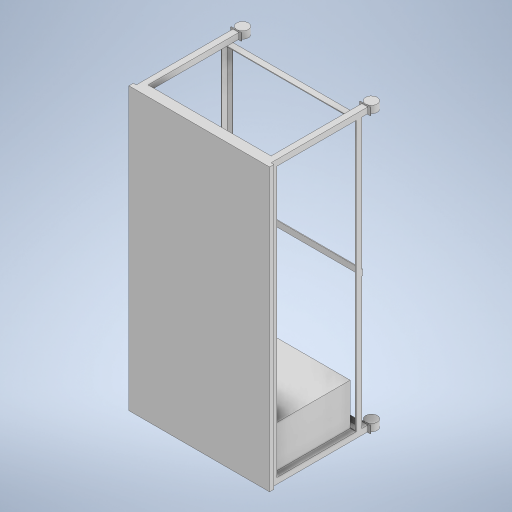
# Autodesk Inventor part: Table Model
Saved by Autodesk Inventor 2023 (Build 270158000, 158)
## iProperties
Created: 2022-09-16
Part Number: Table Model
Material: Generic
Document SubType Name: Modeling
Designer: mikep
Density: 1 g/cm^3
Appearance: Default
Mass: 146789 g
Surface Area: 91872.9 cm^2
Volume: 146789 cm^3
Author: mikep
Autodesk Inventor part; units mm, degrees
ref_plane "YZ Plane" through (0, 0, 0) normal (1, 0, 0) x (0, 1, 0)
ref_plane "XZ Plane" through (0, 0, 0) normal (0, 1, 0) x (-1, 0, 0)
ref_plane "XY Plane" through (0, 0, 0) normal (0, 0, 1) x (1, 0, 0)
sketch "Sketch1" plane through (0, 0, 0) normal (0, 0, 1) x (1, 0, 0)
  line L0 (0, 0) -> (1219.2, 0)
  line L1 (1219.2, 0) -> (1219.2, 2438.4)
  line L2 (1219.2, 2438.4) -> (0, 2438.4)
  line L3 (0, 2438.4) -> (0, 0)
  line L4 (609.6, 0) -> (609.6, 2438.4)
  dimension "d0" = 1219.2
  constraints: 10 end point, 2 midpoint, 2 parallel, 1 horizontal, 1 perpendicular
  measures "d0" distance of L2.end L1.end
extrude "Extrusion1" add sketch "Sketch1" along normal blind 38.1
sketch "Sketch2" plane through (0, 0, 0) normal (0, 0, -1) x (-1, 0, 0)
  line L0 (0, 2438.4) -> (0, 0) projected
  line L1 (-1219.2, 2438.4) -> (0, 2438.4) projected
  line L2 (0, 0) -> (0, 2438.4)
  line L3 (0, 2438.4) -> (-1219.2, 2438.4)
  line L4 (-1219.2, 0) -> (-1219.2, 2438.4) projected
  line L5 (-1219.2, 2438.4) -> (-1219.2, 0)
  line L6 (0, 0) -> (-1219.2, 0) projected
  line L7 (-1219.2, 0) -> (0, 0)
  line L8 (-76.2, 50.8) -> (-1143, 50.8)
  line L9 (-76.2, 50.8) -> (-76.2, 2387.6)
  line L10 (-76.2, 2387.6) -> (-1143, 2387.6)
  line L11 (-1143, 2387.6) -> (-1143, 50.8)
  line L12 (-76.2, 1193.8) -> (-1143, 1193.8)
  line L13 (-1143, 1244.6) -> (-76.2, 1244.6)
  line L14 (-25.4, 0) -> (-25.4, 2438.4)
  line L15 (-1193.8, 2438.4) -> (-1193.8, 0)
  point P0 (-609.6, 0)
  point P1 (-1193.8, 0)
  point P2 (-25.4, 2438.4)
  dimension "d4" = 50.8
  dimension "d5" = 1066.8
  dimension "d8" = 50.8
  dimension "d9" = 1193.8
  dimension "d11" = 50.8
  dimension "d13" = 25.4
  dimension "d19" = 50.8
  constraints: 24 end point, 8 point on line, 6 perpendicular, 3 collinear, 2 parallel, 1 midpoint, 1 vertical
  measures "d4" distance between parallel lines of L6 L8
  measures "d5" distance of L9.end L10.end
  measures "d8" distance between parallel lines of L12 L13
  measures "d9" distance from line of point (-609.6, 0) L12
  measures "d11" distance between parallel lines of L9 L14
  measures "d13" distance between parallel lines of L0 L14
  measures "d19" distance between parallel lines of L1 L10
extrude "Extrusion2" add sketch "Sketch2" along normal blind 50.8 contours L14 L6 L15 L1 | L12 L11 L13 L9
sketch "Sketch3" plane through (0, 0, -50.8) normal (0, 0, -1) x (-1, 0, 0)
  line L0 (-25.4, 2438.4) -> (-25.4, 0) projected
  line L1 (-76.2, 50.8) -> (-25.4, 50.8)
  line L2 (-25.4, 50.8) -> (-25.4, 0)
  line L3 (-25.4, 0) -> (-76.2, 0)
  line L4 (-76.2, 0) -> (-76.2, 50.8)
  line L5 (-1193.8, 0) -> (-25.4, 0) projected
  line L6 (-1143, 1193.8) -> (-1143, 50.8) projected
  line L7 (-1193.8, 0) -> (-1143, 0)
  line L8 (-1143, 0) -> (-1143, 50.8)
  line L9 (-1143, 50.8) -> (-1193.8, 50.8)
  line L10 (-1193.8, 50.8) -> (-1193.8, 0)
  line L11 (-1143, 2387.6) -> (-76.2, 2387.6) projected
  line L12 (-1143, 2387.6) -> (-1193.8, 2387.6)
  line L13 (-1193.8, 2387.6) -> (-1193.8, 2438.4)
  line L14 (-1193.8, 2438.4) -> (-1143, 2438.4)
  line L15 (-1143, 2438.4) -> (-1143, 2387.6)
  line L16 (-1219.2, 2438.4) -> (0, 2438.4) projected
  line L17 (-76.2, 2387.6) -> (-25.4, 2387.6)
  line L18 (-25.4, 2387.6) -> (-25.4, 2438.4)
  line L19 (-25.4, 2438.4) -> (-76.2, 2438.4)
  line L20 (-76.2, 2438.4) -> (-76.2, 2387.6)
  line L21 (-76.2, 1193.8) -> (-1143, 1193.8) projected
  point P0 (0, 0)
  point P1 (-25.4, 1244.6)
  dimension "d18" = 50.8
  constraints: 32 end point, 8 parallel, 6 point on line, 4 horizontal, 4 perpendicular
  measures "d18" distance of L14.end L11.start
extrude "Extrusion3" add sketch "Sketch3" along normal blind 736.6 contours L5 L10 L9 L8 | L0 L3 L4 L1 | L0 L17 L20 L16 | L15 L12 L13 L14
sketch "Sketch8" plane through (25.4, 2387.6, -50.8) normal (0, -1, 0) x (1, 0, 0)
  line L0 (0, -735.9482) -> (0, -685.1482)
  line L1 (0, 0) -> (0, -736.6) projected
  line L2 (0, -685.1482) -> (6.35, -685.1482)
  line L3 (50.8, -736.6) -> (0, -736.6) projected
  line L4 (0, -736.6) -> (50.8, -736.6)
  line L5 (50.8, -736.6) -> (50.8, -730.25)
  line L6 (50.8, 0) -> (50.8, -736.6) projected
  line L7 (50.8, -730.25) -> (6.35, -730.25)
  line L8 (6.35, -730.25) -> (6.35, -685.1482)
  line L9 (1168.4, 0) -> (1168.4, -736.6) projected
  line L10 (1168.4, -736.6) -> (1168.4, -685.8)
  line L11 (1168.4, -685.8) -> (1168.4, -736.6)
  line L12 (1168.4, -736.6) -> (1117.6, -736.6) projected
  line L13 (1168.4, -736.6) -> (1117.6, -736.6)
  line L14 (1117.6, -736.6) -> (1117.6, -730.25)
  line L15 (1117.6, 0) -> (1117.6, -736.6) projected
  line L16 (1117.6, -730.25) -> (1162.05, -730.25)
  line L17 (1162.05, -730.25) -> (1162.05, -685.8)
  line L18 (1162.05, -685.8) -> (1168.4, -685.8)
  point P0 (-25.4, 50.8)
  point P1 (0, -735.9482)
  dimension "d40" = 50.8
  dimension "d41" = 6.35
  dimension "d42" = 6.35
  dimension "d43" = 44.45
  dimension "d44" = 50.8
  dimension "d45" = 6.35
  dimension "d46" = 44.45
  dimension "d47" = 44.45
  constraints: 26 end point, 5 perpendicular, 4 point on line, 2 horizontal, 1 collinear
  measures "d40" distance of L0.start L0.end
  measures "d41" distance of L0.end L2.end
  measures "d42" distance of L3.start L5.end
  measures "d43" distance of L5.end L7.end
  measures "d44" distance of L9.end L10.end
  measures "d45" distance of L12.end L14.end
  measures "d46" distance of L14.end L16.end
  measures "d47" distance of L16.end L17.end
extrude "Extrusion6" add sketch "Sketch8" along normal blind 2336.8
sketch "Sketch9" plane through (1187.45, 50.8, -781.05) normal (-1, 0, 0) x (0, 0, 1)
  line L0 (44.45, 0) -> (0, 0) projected
  line L1 (44.45, 0) -> (44.45, 6.35)
  line L2 (44.45, 2336.8) -> (44.45, 0) projected
  line L3 (44.45, 6.35) -> (0, 6.35)
  line L4 (0, 2336.8) -> (0, 0) projected
  line L5 (44.45, 2336.8) -> (44.45, 0) projected
  line L6 (0, 0) -> (44.45, 0)
  line L7 (0, 2336.8) -> (44.45, 2336.8) projected
  line L8 (44.45, 2336.8) -> (0, 2336.8)
  line L9 (0, 2336.8) -> (0, 2330.45)
  line L10 (0, 2330.45) -> (44.45, 2330.45)
  point P0 (781.05, -50.8)
  dimension "d50" = 6.35
  dimension "d51" = 6.35
  constraints: 12 end point, 4 point on line, 2 perpendicular, 1 collinear, 1 horizontal
  measures "d50" distance of L0.start L1.end
  measures "d51" distance of L4.start L9.end
extrude "Extrusion7" add sketch "Sketch9" along normal blind 1155.7 contours L0 L4 L3 L1 | L10 L4 L7 L2
sketch "Sketch10" plane through (76.2, 0, -787.4) normal (1, 0, 0) x (0, 0, -1)
  line L0 (-6.35, 2387.6) -> (-6.35, 2381.25) projected
  line L1 (-6.35, 2387.6) -> (-6.35, 2336.8)
  line L2 (-6.35, 2381.25) -> (-6.35, 57.15) projected
  line L3 (-6.35, 2336.8) -> (0, 2336.8)
  line L4 (0, 2438.4) -> (0, 0) projected
  line L5 (0, 2387.6) -> (-6.35, 2387.6)
  line L6 (-6.35, 50.8) -> (0, 50.8)
  line L7 (0, 50.8) -> (0, 101.6)
  line L8 (0, 0) -> (0, 2438.4) projected
  line L9 (0, 101.6) -> (-6.35, 101.6)
  line L10 (-6.35, 101.6) -> (-6.35, 50.8)
  point P0 (-787.4, 0)
  dimension "d54" = 50.8
  dimension "d55" = 50.8
  constraints: 14 end point, 5 point on line, 4 perpendicular, 1 horizontal
  measures "d54" distance of L0.start L1.end
  measures "d55" distance of L6.end L7.end
extrude "Extrusion8" add sketch "Sketch10" along normal blind 1066.8 contours L5 L4 L3 L1 L0 | L9 L4 L6 L10 L2
sketch "Sketch12" plane through (0, 0, -787.4) normal (0, 0, -1) x (-1, 0, 0)
  line L0 (-1143, 1193.8) -> (-76.2, 1193.8) projected
  line L1 (-76.2, 1193.8) -> (-25.4, 1193.8)
  line L2 (-25.4, 50.8) -> (-25.4, 2387.6) projected
  line L3 (-25.4, 1193.8) -> (-25.4, 1244.6)
  line L4 (-25.4, 2387.6) -> (-25.4, 50.8) projected
  line L5 (-25.4, 1244.6) -> (-76.2, 1244.6)
  line L6 (-76.2, 2336.8) -> (-76.2, 101.6) projected
  line L7 (-76.2, 1193.8) -> (-76.2, 1244.6)
  line L8 (-76.2, 2336.8) -> (-76.2, 101.6) projected
  point P0 (0, 0)
  dimension "d58" = 50.8
  constraints: 8 end point, 3 point on line, 1 collinear, 1 horizontal, 1 perpendicular
  measures "d58" distance of L1.end L3.end
extrude "Extrusion9" add sketch "Sketch12" along normal blind 6.35
sketch "Sketch13" plane through (76.2, 101.6, -781.05) normal (1, 0, 0) x (0, 0, -1)
  line L0 (6.35, 1092.2) -> (6.35, 0) projected
  line L1 (6.35, 2235.2) -> (6.35, 1143) projected
  line L2 (6.35, 1092.2) -> (6.35, 1143)
  line L3 (6.35, 1143) -> (12.7, 1143) projected
  line L4 (6.35, 1143) -> (12.7, 1143)
  line L5 (12.7, 1143) -> (12.7, 1092.2)
  line L6 (6.35, 1092.2) -> (12.7, 1092.2) projected
  line L7 (12.7, 1092.2) -> (6.35, 1092.2)
  point P0 (-781.05, -101.6)
  constraints: 8 end point, 2 perpendicular, 1 collinear, 1 vertical
extrude "Extrusion10" add sketch "Sketch13" along normal blind 1117.6
sketch "Sketch14" plane through (0, 0, -787.4) normal (0, 0, -1) x (-1, 0, 0)
  line L0 (-25.4, 0) -> (-25.4, 1193.8) projected
  line L1 (-76.2, 50.8) -> (-76.2, 0) projected
  line L2 (-25.4, 0) -> (-76.2, 0)
  line L3 (-76.2, 0) -> (-76.2, 50.8)
  line L4 (-76.2, 50.8) -> (-25.4, 50.8) projected
  line L5 (-76.2, 50.8) -> (-25.4, 50.8)
  line L6 (-25.4, 50.8) -> (-25.4, 0)
  line L7 (-1193.8, 0) -> (-1143, 0) projected
  line L8 (-1193.8, 2387.6) -> (-1193.8, 50.8) projected
  line L9 (-1143, 0) -> (-1193.8, 0)
  line L10 (-1193.8, 0) -> (-1193.8, 50.8)
  line L11 (-1193.8, 50.8) -> (-1143, 50.8)
  line L12 (-1143, 50.8) -> (-1143, 0)
  line L13 (-1143, 2387.6) -> (-1143, 2438.4) projected
  line L14 (-1143, 2387.6) -> (-1193.8, 2387.6)
  line L15 (-1193.8, 2387.6) -> (-1193.8, 2438.4)
  line L16 (-1193.8, 2438.4) -> (-1143, 2438.4)
  line L17 (-1143, 2438.4) -> (-1143, 2387.6)
  line L18 (-76.2, 2387.6) -> (-1143, 2387.6) projected
  line L19 (-25.4, 2438.4) -> (-25.4, 0) projected
  line L20 (-76.2, 2387.6) -> (-25.4, 2387.6)
  line L21 (-25.4, 2387.6) -> (-25.4, 2438.4)
  line L22 (-25.4, 2438.4) -> (-76.2, 2438.4)
  line L23 (-76.2, 2438.4) -> (-76.2, 2387.6)
  point P0 (0, 0)
  constraints: 32 end point, 8 equal length, 4 horizontal, 4 perpendicular
extrude "Extrusion11" add sketch "Sketch14" along normal blind 50.8
sketch "Sketch15" plane through (0, 0, -50.8) normal (0, 0, -1) x (-1, 0, 0)
  line L0 (-76.2, 2387.6) -> (-76.2, 1244.6) projected
  line L1 (-25.4, 2387.6) -> (-76.2, 2387.6) projected
  line L2 (-1193.8, 2387.6) -> (-1193.8, 50.8) projected
  line L3 (-1143, 2387.6) -> (-1193.8, 2387.6) projected
  line L4 (-1143, 50.8) -> (-1143, 1193.8) projected
  line L5 (-1193.8, 50.8) -> (-1143, 50.8) projected
  line L6 (-25.4, 50.8) -> (-25.4, 2387.6) projected
  line L7 (-76.2, 50.8) -> (-25.4, 50.8) projected
  line L8 (-1143, 1193.8) -> (-76.2, 1193.8) projected
  line L9 (-76.2, 2438.4) -> (-1143, 2438.4) projected
  line L10 (-1143, 2438.4) -> (-1143, 2387.6) projected
  line L11 (-76.2, 2387.6) -> (-76.2, 2438.4) projected
  point P0 (0, 0)
  point P1 (-50.8, 2336.8)
  point P2 (-50.8, 2387.6)
  point P3 (-1168.4, 2336.8)
  point P4 (-1168.4, 101.6)
  point P5 (-1168.4, 50.8)
  point P6 (-50.8, 101.6)
  point P7 (-50.8, 1219.2)
  point P8 (-1168.4, 1219.2)
  point P9 (-1193.8, 1219.2)
  point P10 (-1092.2, 2413)
  point P11 (-1143, 2413)
  point P12 (-127, 2413)
  point P13 (-127, 26.9736)
  point P14 (-1092.2, 24.7592)
  dimension "d65" = 25.4
  dimension "d66" = 50.8
  dimension "d67" = 25.4
  dimension "d68" = 50.8
  dimension "d69" = 25.4
  dimension "d70" = 50.8
  dimension "d71" = 25.4
  dimension "d72" = 50.8
  dimension "d80" = 25.4
  dimension "d81" = 25.4
  dimension "d82" = 25.4
  dimension "d83" = 50.8
  dimension "d84" = 50.8
  constraints: 4 midpoint
  measures "d65" distance from line of L0 point (-50.8, 2336.8)
  measures "d66" distance of point (-50.8, 2387.6) point (-50.8, 2336.8)
  measures "d67" distance from line of L2 point (-1168.4, 2336.8)
  measures "d68" distance from line of L3 point (-1168.4, 2336.8)
  measures "d69" distance from line of L4 point (-1168.4, 101.6)
  measures "d70" distance of point (-1168.4, 50.8) point (-1168.4, 101.6)
  measures "d71" distance from line of L6 point (-50.8, 101.6)
  measures "d72" distance from line of L7 point (-50.8, 101.6)
  measures "d80" distance of point (-1193.8, 1219.2) point (-1168.4, 1219.2)
  measures "d81" distance from line of L8 point (-1168.4, 1219.2)
  measures "d82" distance from line of L9 point (-1092.2, 2413)
  measures "d83" distance of point (-1143, 2413) point (-1092.2, 2413)
  measures "d84" distance from line of L11 point (-127, 2413)
hole "Hole1" at (50.8, 2336.8, -50.8) at (1168.4, 2336.8, -50.8) at (1168.4, 101.6, -50.8) at (50.8, 101.6, -50.8) direction (0, 0, 1) diameter 8.255 depth 19.05 tip angle 118
sketch "Sketch16" plane through (0, 0, -838.2) normal (0, 0, -1) x (-1, 0, 0)
  line L0 (-4.826, -5.588) -> (-96.774, -5.588)
  line L1 (-96.774, -5.588) -> (-96.774, 56.388)
  line L2 (-96.774, 56.388) -> (-4.826, 56.388)
  line L3 (-4.826, 56.388) -> (-4.826, -5.588)
  line L4 (-76.2, 50.8) -> (-76.2, 0) projected
  line L5 (-1122.426, -5.588) -> (-1214.374, -5.588)
  line L6 (-1214.374, -5.588) -> (-1214.374, 56.388)
  line L7 (-1214.374, 56.388) -> (-1122.426, 56.388)
  line L8 (-1122.426, 56.388) -> (-1122.426, -5.588)
  line L9 (-1143, 0) -> (-1143, 50.8) projected
  line L10 (-1193.8, 0) -> (-1143, 0) projected
  line L11 (-76.2, 0) -> (-25.4, 0) projected
  line L12 (-96.774, 2443.988) -> (-4.826, 2443.988)
  line L13 (-4.826, 2443.988) -> (-4.826, 2382.012)
  line L14 (-4.826, 2382.012) -> (-96.774, 2382.012)
  line L15 (-96.774, 2382.012) -> (-96.774, 2443.988)
  line L16 (-76.2, 2387.6) -> (-25.4, 2387.6) projected
  line L17 (-76.2, 2438.4) -> (-76.2, 2387.6) projected
  line L18 (-1122.426, 2382.012) -> (-1214.374, 2382.012)
  line L19 (-1214.374, 2382.012) -> (-1214.374, 2443.988)
  line L20 (-1214.374, 2443.988) -> (-1122.426, 2443.988)
  line L21 (-1122.426, 2443.988) -> (-1122.426, 2382.012)
  line L22 (-1193.8, 2438.4) -> (-1193.8, 2387.6) projected
  line L23 (-1193.8, 2387.6) -> (-1143, 2387.6) projected
  point P0 (0, 0)
  point P1 (-50.8, -5.588)
  point P2 (-76.2, 2413)
  point P3 (-96.774, 2413)
  dimension "d85" = 91.948
  dimension "d86" = 61.976
  dimension "d88" = 61.976
  dimension "d89" = 91.948
  dimension "d90" = 20.574
  dimension "d91" = 5.588
  dimension "d92" = 5.588
  dimension "d93" = 61.976
  dimension "d94" = 91.948
  dimension "d95" = 5.588
  dimension "d96" = 20.574
  dimension "d97" = 61.976
  dimension "d98" = 91.948
  dimension "d99" = 20.574
  dimension "d100" = 5.588
  constraints: 32 end point, 8 parallel, 4 horizontal, 4 perpendicular, 3 midpoint
  measures "d85" distance of L0.start L0.end
  measures "d86" distance of L2.end L0.start
  measures "d88" distance of L5.end L6.end
  measures "d89" distance of L6.end L7.end
  measures "d90" distance between parallel lines of L8 L9
  measures "d91" distance between parallel lines of L10 L5
  measures "d92" distance from line of L11 point (-50.8, -5.588)
  measures "d93" distance of L12.end L13.end
  measures "d94" distance of L13.end L14.end
  measures "d95" distance between parallel lines of L16 L14
  measures "d96" distance of point (-76.2, 2413) point (-96.774, 2413)
  measures "d97" distance of L18.end L19.end
  measures "d98" distance of L18.start L18.end
  measures "d99" distance between parallel lines of L22 L19
  measures "d100" distance between parallel lines of L23 L18
extrude "Extrusion12" add sketch "Sketch16" along normal blind 6.35
sketch "Sketch17" plane through (4.826, 2382.012, -838.2) normal (0, -1, 0) x (1, 0, 0)
  line L0 (91.948, -6.35) -> (0, -6.35) projected
  circle A0 centre (45.974, -57.15) radius 50.8
  circle A1 centre (1163.574, -57.15) radius 50.8
  point P0 (-4.826, 838.2)
  point P1 (45.974, -6.35)
  dimension "d104" = 101.6
  dimension "d105" = 50.8
  constraints: 2 centre point, 1 midpoint
  measures "d104" diameter of A0
  measures "d105" distance of A0.centre point (45.974, -6.35)
extrude "Extrusion13" add sketch "Sketch17" against normal blind 61.976
sketch "Sketch18" plane through (4.826, -5.588, -838.2) normal (0, -1, 0) x (1, 0, 0)
  circle A0 centre (44.7722, -57.0272) radius 50.8
  circle A1 centre (1163.9993, -57.0272) radius 50.8
  point P0 (-4.826, 838.2)
  dimension "d108" = 101.6
  dimension "d109" = 101.6
  constraints: 2 centre point
  measures "d108" diameter of A0
  measures "d109" diameter of A1
extrude "Extrusion14" add sketch "Sketch18" against normal blind 61.976
sketch "Sketch19" plane through (0, 0, 38.1) normal (0, -1, 0) x (1, 0, 0)
  line L0 (76.2, -88.9) -> (76.2, -876.3) projected
  line L1 (76.2, -88.9) -> (1143, -88.9)
  line L2 (1143, -88.9) -> (1143, -774.7)
  line L3 (1143, -774.7) -> (76.2, -774.7)
  line L4 (76.2, -774.7) -> (76.2, -88.9)
  line L5 (82.55, -95.25) -> (1136.65, -95.25)
  line L6 (1136.65, -95.25) -> (1136.65, -768.35)
  line L7 (1136.65, -768.35) -> (82.55, -768.35)
  line L8 (82.55, -768.35) -> (82.55, -95.25)
  point P0 (0, -38.1)
  point P1 (76.2, -774.7)
  dimension "d112" = 1066.8
  dimension "d113" = 685.8
  dimension "d114" = 6.35
  dimension "d115" = 6.35
  dimension "d116" = 6.35
  dimension "d117" = 6.35
  constraints: 16 end point, 4 parallel, 2 horizontal, 2 perpendicular
  measures "d112" distance of L2.end L3.end
  measures "d113" distance of L1.end L2.end
  measures "d114" distance between parallel lines of L2 L6
  measures "d115" distance between parallel lines of L3 L7
  measures "d116" distance between parallel lines of L0 L8
  measures "d117" distance between parallel lines of L1 L5
extrude "Extrusion15" add sketch "Sketch19" against normal blind 406.4
sketch "Sketch20" plane through (0, 406.4, 38.1) normal (0, 1, 0) x (1, 0, 0)
  line L0 (76.2, 774.7) -> (76.2, 88.9) projected
  line L1 (1143, 88.9) -> (1143, 774.7) projected
  line L2 (76.2, 88.9) -> (1143, 88.9)
  line L3 (1143, 88.9) -> (1143, 774.7)
  line L4 (1143, 774.7) -> (76.2, 774.7)
  line L5 (76.2, 774.7) -> (76.2, 88.9)
  point P0 (0, 38.1)
  constraints: 8 end point, 2 parallel, 1 horizontal, 1 perpendicular
extrude "Extrusion16" add sketch "Sketch20" along normal blind 6.35
sketch "Sketch21" plane through (0, 406.4, 38.1) normal (0, -1, 0) x (1, 0, 0)
  line L0 (1136.65, -95.25) -> (82.55, -95.25) projected
  line L1 (82.55, -768.35) -> (1136.65, -768.35) projected
  line L2 (514.35, -95.25) -> (520.7, -95.25)
  line L3 (520.7, -95.25) -> (520.7, -768.35)
  line L4 (520.7, -768.35) -> (514.35, -768.35)
  line L5 (514.35, -768.35) -> (514.35, -95.25)
  line L6 (82.55, -768.35) -> (82.55, -95.25) projected
  line L7 (82.55, -95.25) -> (1136.65, -95.25) projected
  line L8 (76.2, -774.7) -> (1143, -774.7) projected
  line L9 (952.5, -95.25) -> (958.85, -95.25)
  line L10 (958.85, -95.25) -> (958.85, -774.7)
  line L11 (958.85, -774.7) -> (952.5, -774.7)
  line L12 (952.5, -774.7) -> (952.5, -95.25)
  line L13 (1136.65, -768.35) -> (1136.65, -95.25) projected
  line L14 (82.55, -95.25) -> (82.55, -768.35) projected
  line L15 (82.55, -222.25) -> (514.35, -222.25)
  line L16 (514.35, -222.25) -> (514.35, -228.6)
  line L17 (514.35, -228.6) -> (82.55, -228.6)
  line L18 (82.55, -228.6) -> (82.55, -222.25)
  line L19 (520.7, -222.25) -> (952.5, -222.25)
  line L20 (952.5, -222.25) -> (952.5, -228.6)
  line L21 (952.5, -228.6) -> (520.7, -228.6)
  line L22 (520.7, -228.6) -> (520.7, -222.25)
  line L23 (1136.65, -95.25) -> (1136.65, -768.35) projected
  line L24 (958.85, -228.6) -> (1136.65, -228.6)
  line L25 (1136.65, -228.6) -> (1136.65, -222.25)
  line L26 (1136.65, -222.25) -> (958.85, -222.25)
  line L27 (958.85, -222.25) -> (958.85, -228.6)
  line L28 (82.55, -355.6) -> (514.35, -355.6)
  line L29 (514.35, -355.6) -> (514.35, -361.95)
  line L30 (514.35, -361.95) -> (82.55, -361.95)
  line L31 (82.55, -361.95) -> (82.55, -355.6)
  line L32 (520.7, -361.95) -> (952.5, -361.95)
  line L33 (952.5, -361.95) -> (952.5, -355.6)
  line L34 (952.5, -355.6) -> (520.7, -355.6)
  line L35 (520.7, -355.6) -> (520.7, -361.95)
  line L36 (958.85, -355.6) -> (1136.65, -355.6)
  line L37 (1136.65, -355.6) -> (1136.65, -361.95)
  line L38 (1136.65, -361.95) -> (958.85, -361.95)
  line L39 (958.85, -361.95) -> (958.85, -355.6)
  line L40 (82.55, -488.95) -> (514.35, -488.95)
  line L41 (514.35, -488.95) -> (514.35, -495.3)
  line L42 (514.35, -495.3) -> (82.55, -495.3)
  line L43 (82.55, -495.3) -> (82.55, -488.95)
  line L44 (520.7, -488.95) -> (952.5, -488.95)
  line L45 (952.5, -488.95) -> (952.5, -495.3)
  line L46 (952.5, -495.3) -> (520.7, -495.3)
  line L47 (520.7, -495.3) -> (520.7, -488.95)
  line L48 (958.85, -495.3) -> (1136.65, -495.3)
  line L49 (1136.65, -495.3) -> (1136.65, -488.95)
  line L50 (1136.65, -488.95) -> (958.85, -488.95)
  line L51 (958.85, -488.95) -> (958.85, -495.3)
  line L52 (82.55, -628.5398) -> (514.35, -628.5398)
  line L53 (514.35, -628.5398) -> (514.35, -622.1898)
  line L54 (514.35, -622.1898) -> (82.55, -622.1898)
  line L55 (82.55, -622.1898) -> (82.55, -628.5398)
  line L56 (520.7, -628.5398) -> (952.5, -628.5398)
  line L57 (952.5, -628.5398) -> (952.5, -622.1898)
  line L58 (952.5, -622.1898) -> (520.7, -622.1898)
  line L59 (520.7, -622.1898) -> (520.7, -628.5398)
  line L60 (958.85, -628.5398) -> (1136.65, -628.5398)
  line L61 (1136.65, -628.5398) -> (1136.65, -622.1898)
  line L62 (1136.65, -622.1898) -> (958.85, -622.1898)
  line L63 (958.85, -622.1898) -> (958.85, -628.5398)
  point P0 (0, -38.1)
  point P1 (958.85, -434.975)
  point P2 (1047.75, -355.6)
  point P3 (82.55, -228.6)
  point P4 (82.55, -361.95)
  point P5 (82.55, -495.3)
  point P6 (82.55, -622.1898)
  point P7 (1136.65, -361.95)
  dimension "d122" = 6.35
  dimension "d123" = 431.8
  dimension "d124" = 6.35
  dimension "d126" = 431.8
  dimension "d127" = 6.35
  dimension "d128" = 127
  dimension "d129" = 6.35
  dimension "d130" = 127
  dimension "d131" = 127
  dimension "d132" = 431.8
  dimension "d133" = 6.35
  dimension "d134" = 127
  dimension "d135" = 6.35
  constraints: 112 end point, 38 point on line, 28 parallel, 14 horizontal, 14 perpendicular, 2 midpoint
  measures "d122" distance of L3.end L4.end
  measures "d123" distance between parallel lines of L6 L5
  measures "d124" distance from line of point (958.85, -434.975) L12
  measures "d126" distance between parallel lines of L3 L12
  measures "d127" distance between parallel lines of L15 L17
  measures "d128" distance between parallel lines of L0 L15
  measures "d129" distance of L28.end L29.end
  measures "d130" distance between parallel lines of L28 L17
  measures "d131" distance from line of point (1047.75, -355.6) L24
  measures "d132" distance of L41.end L42.end
  measures "d133" distance of L40.end L41.end
  measures "d134" distance between parallel lines of L40 L30
  measures "d135" distance of L53.end L52.end
extrude "Extrusion17" add sketch "Sketch21" along normal blind 406.4 contours L10 L1 L12 L0 | L13 L24 L10 L26 | L3 L1 L5 L0 | L12 L21 L3 L19 | L13 L38 L10 L36 | L5 L17 L6 L15 | L12 L32 L3 L34 | L13 L48 L10 L50 | L5 L30 L6 L28 | L12 L46 L3 L44 | L13 L60 L10 L62 | L5 L42 L6 L40 | L12 L56 L3 L58 | L10 L8 L12 L1 | L5 L52 L6 L54
sketch "Sketch22" plane through (82.55, 406.4, -184.15) normal (0, 0, 1) x (1, 0, 0)
  line L0 (0, -406.4) -> (142.24, -406.4)
  line L1 (142.24, -406.4) -> (142.24, -400.05)
  line L2 (142.24, -400.05) -> (0, -400.05)
  line L3 (0, -400.05) -> (0, -406.4)
  line L4 (431.8, 0) -> (431.8, -406.4) projected
  line L5 (431.8, -406.4) -> (289.56, -406.4)
  line L6 (289.56, -406.4) -> (289.56, -400.05)
  line L7 (289.56, -400.05) -> (431.8, -400.05)
  line L8 (431.8, -400.05) -> (431.8, -406.4)
  line L9 (438.15, 0) -> (438.15, -406.4) projected
  line L10 (438.15, -406.4) -> (580.39, -406.4)
  line L11 (580.39, -406.4) -> (580.39, -400.05)
  line L12 (580.39, -400.05) -> (438.15, -400.05)
  line L13 (438.15, -400.05) -> (438.15, -406.4)
  line L14 (869.95, -406.4) -> (727.71, -406.4)
  line L15 (727.71, -406.4) -> (727.71, -400.05)
  line L16 (727.71, -400.05) -> (869.95, -400.05)
  line L17 (869.95, -400.05) -> (869.95, -406.4)
  line L18 (876.3, -406.4) -> (1054.1, -406.4) projected
  line L19 (876.3, -406.4) -> (934.72, -406.4)
  line L20 (934.72, -406.4) -> (934.72, -401.32)
  line L21 (934.72, -401.32) -> (876.3, -401.32)
  line L22 (876.3, -401.32) -> (876.3, -406.4)
  line L23 (1054.1, -406.4) -> (1054.1, 0) projected
  line L24 (1054.1, -406.4) -> (995.68, -406.4)
  line L25 (995.68, -406.4) -> (995.68, -400.05)
  line L26 (995.68, -400.05) -> (1054.1, -400.05)
  line L27 (1054.1, -400.05) -> (1054.1, -406.4)
  point P0 (-82.55, -406.4)
  dimension "d138" = 142.24
  dimension "d139" = 6.35
  dimension "d140" = 142.24
  dimension "d141" = 6.35
  dimension "d144" = 142.24
  dimension "d145" = 6.35
  dimension "d146" = 142.24
  dimension "d147" = 6.35
  dimension "d148" = 58.42
  dimension "d149" = 5.08
  dimension "d150" = 58.42
  dimension "d151" = 6.35
  constraints: 48 end point, 12 parallel, 6 horizontal, 6 perpendicular
  measures "d138" distance of L2.end L1.end
  measures "d139" distance between parallel lines of L0 L2
  measures "d140" distance of L6.end L7.end
  measures "d141" distance of L5.end L6.end
  measures "d144" distance of L12.end L11.end
  measures "d145" distance of L11.end L10.end
  measures "d146" distance of L15.end L16.end
  measures "d147" distance of L14.end L15.end
  measures "d148" distance of L21.end L20.end
  measures "d149" distance of L20.end L19.end
  measures "d150" distance of L25.end L26.end
  measures "d151" distance of L24.end L25.end
extrude "Extrusion18" add sketch "Sketch22" along normal blind 6.35 contours L3 L2 L1 L0 | L4 L5 L6 L7
extrude "Extrusion19" add sketch "Sketch22" along normal blind 6.35 contours L12 L11 L10 L9 | L14 L15 L16 L17 | L22 L21 L20 L18 | L25 L26 L23 L18
sketch "Sketch23" plane through (82.55, 406.4, -317.5) normal (0, 0, 1) x (1, 0, 0)
  line L0 (0, 0) -> (0, -406.4) projected
  line L1 (0, -406.4) -> (142.24, -406.4)
  line L2 (142.24, -406.4) -> (142.24, -400.05)
  line L3 (142.24, -400.05) -> (0, -400.05)
  line L4 (0, -400.05) -> (0, -406.4)
  line L5 (431.8, -406.4) -> (289.56, -406.4)
  line L6 (289.56, -406.4) -> (289.56, -400.05)
  line L7 (289.56, -400.05) -> (431.8, -400.05)
  line L8 (431.8, -400.05) -> (431.8, -406.4)
  line L9 (438.15, -406.4) -> (580.39, -406.4)
  line L10 (580.39, -406.4) -> (580.39, -400.05)
  line L11 (580.39, -400.05) -> (438.15, -400.05)
  line L12 (438.15, -400.05) -> (438.15, -406.4)
  line L13 (438.15, -406.4) -> (869.95, -406.4) projected
  line L14 (869.95, -406.4) -> (727.71, -406.4)
  line L15 (727.71, -406.4) -> (727.71, -400.05)
  line L16 (727.71, -400.05) -> (869.95, -400.05)
  line L17 (869.95, -400.05) -> (869.95, -406.4)
  line L18 (1054.1, -406.4) -> (876.3, -406.4) projected
  line L19 (876.3, -406.4) -> (934.72, -406.4)
  line L20 (934.72, -406.4) -> (934.72, -400.05)
  line L21 (934.72, -400.05) -> (876.3, -400.05)
  line L22 (876.3, -400.05) -> (876.3, -406.4)
  line L23 (1054.1, -406.4) -> (995.68, -406.4)
  line L24 (995.68, -406.4) -> (995.68, -400.05)
  line L25 (995.68, -400.05) -> (1054.1, -400.05)
  line L26 (1054.1, -400.05) -> (1054.1, -406.4)
  point P0 (-82.55, -406.4)
  point P1 (0, -400.05)
  dimension "d154" = 142.24
  dimension "d155" = 6.35
  dimension "d156" = 142.24
  dimension "d157" = 6.35
  dimension "d158" = 142.24
  dimension "d159" = 6.35
  dimension "d160" = 142.24
  dimension "d161" = 6.35
  dimension "d162" = 58.42
  dimension "d163" = 6.35
  dimension "d164" = 58.42
  constraints: 48 end point, 12 parallel, 6 horizontal, 6 perpendicular, 1 point on line
  measures "d154" distance of L3.end L2.end
  measures "d155" distance of L2.end L1.end
  measures "d156" distance of L6.end L7.end
  measures "d157" distance of L5.end L6.end
  measures "d158" distance of L11.end L10.end
  measures "d159" distance of L10.end L9.end
  measures "d160" distance of L15.end L16.end
  measures "d161" distance of L14.end L15.end
  measures "d162" distance of L21.end L20.end
  measures "d163" distance of L20.end L19.end
  measures "d164" distance of L24.end L25.end
extrude "Extrusion20" add sketch "Sketch23" along normal blind 6.35
sketch "Sketch24" plane through (82.55, 406.4, -450.85) normal (0, 0, 1) x (1, 0, 0)
  line L0 (431.8, -406.4) -> (0, -406.4) projected
  line L1 (0, -406.4) -> (142.24, -406.4)
  line L2 (142.24, -406.4) -> (142.24, -400.05)
  line L3 (142.24, -400.05) -> (0, -400.05)
  line L4 (0, -400.05) -> (0, -406.4)
  line L5 (431.8, -406.4) -> (289.56, -406.4)
  line L6 (289.56, -406.4) -> (289.56, -400.05)
  line L7 (289.56, -400.05) -> (431.8, -400.05)
  line L8 (431.8, -400.05) -> (431.8, -406.4)
  line L9 (438.15, -406.4) -> (869.95, -406.4) projected
  line L10 (438.15, -406.4) -> (580.39, -406.4)
  line L11 (580.39, -406.4) -> (580.39, -400.05)
  line L12 (580.39, -400.05) -> (438.15, -400.05)
  line L13 (438.15, -400.05) -> (438.15, -406.4)
  line L14 (869.95, -406.4) -> (727.71, -406.4)
  line L15 (727.71, -406.4) -> (727.71, -400.05)
  line L16 (727.71, -400.05) -> (869.95, -400.05)
  line L17 (869.95, -400.05) -> (869.95, -406.4)
  line L18 (876.3, -406.4) -> (1054.1, -406.4) projected
  line L19 (876.3, -406.4) -> (934.72, -406.4)
  line L20 (934.72, -406.4) -> (934.72, -400.05)
  line L21 (934.72, -400.05) -> (876.3, -400.05)
  line L22 (876.3, -400.05) -> (876.3, -406.4)
  line L23 (1054.1, -406.4) -> (1054.1, 0) projected
  line L24 (1054.1, -406.4) -> (995.68, -406.4)
  line L25 (995.68, -406.4) -> (995.68, -400.05)
  line L26 (995.68, -400.05) -> (1054.1, -400.05)
  line L27 (1054.1, -400.05) -> (1054.1, -406.4)
  point P0 (-82.55, -406.4)
  point P1 (1054.1, -400.05)
  point P2 (995.68, -406.4)
  point P3 (934.72, -406.4)
  point P4 (727.71, -406.4)
  dimension "d167" = 142.24
  dimension "d168" = 6.35
  dimension "d169" = 142.24
  dimension "d170" = 142.24
  dimension "d171" = 142.24
  dimension "d172" = 58.42
  dimension "d173" = 6.35
  dimension "d174" = 58.42
  dimension "d175" = 6.35
  constraints: 48 end point, 12 parallel, 6 horizontal, 6 perpendicular, 2 point on line
  measures "d167" distance of L3.end L2.end
  measures "d168" distance of L2.end L1.end
  measures "d169" distance of L6.end L7.end
  measures "d170" distance of L12.end L11.end
  measures "d171" distance of L15.end L16.end
  measures "d172" distance of L21.end L20.end
  measures "d173" distance of L20.end L19.end
  measures "d174" distance of L25.end L26.end
  measures "d175" distance of L24.end L25.end
extrude "Extrusion21" add sketch "Sketch24" along normal blind 6.35
sketch "Sketch25" plane through (82.55, 406.4, -584.0898) normal (0, 0, 1) x (1, 0, 0)
  line L0 (0, -406.4) -> (142.24, -406.4)
  line L1 (142.24, -406.4) -> (142.24, -400.05)
  line L2 (142.24, -400.05) -> (0, -400.05)
  line L3 (0, -400.05) -> (0, -406.4)
  line L4 (431.8, -406.4) -> (0, -406.4) projected
  line L5 (431.8, -406.4) -> (289.56, -406.4)
  line L6 (289.56, -406.4) -> (289.56, -400.05)
  line L7 (289.56, -400.05) -> (431.8, -400.05)
  line L8 (431.8, -400.05) -> (431.8, -406.4)
  line L9 (869.95, -406.4) -> (438.15, -406.4) projected
  line L10 (438.15, -406.4) -> (580.39, -406.4)
  line L11 (580.39, -406.4) -> (580.39, -400.05)
  line L12 (580.39, -400.05) -> (438.15, -400.05)
  line L13 (438.15, -400.05) -> (438.15, -406.4)
  line L14 (869.95, -406.4) -> (727.71, -406.4)
  line L15 (727.71, -406.4) -> (727.71, -400.05)
  line L16 (727.71, -400.05) -> (869.95, -400.05)
  line L17 (869.95, -400.05) -> (869.95, -406.4)
  line L18 (876.3, -406.4) -> (1054.1, -406.4) projected
  line L19 (876.3, -406.4) -> (934.72, -406.4)
  line L20 (934.72, -406.4) -> (934.72, -400.05)
  line L21 (934.72, -400.05) -> (876.3, -400.05)
  line L22 (876.3, -400.05) -> (876.3, -406.4)
  line L23 (1054.1, -406.4) -> (876.3, -406.4) projected
  line L24 (1054.1, -406.4) -> (995.68, -406.4)
  line L25 (995.68, -406.4) -> (995.68, -400.05)
  line L26 (995.68, -400.05) -> (1054.1, -400.05)
  line L27 (1054.1, -400.05) -> (1054.1, -406.4)
  point P0 (-82.55, -406.4)
  dimension "d178" = 142.24
  dimension "d179" = 6.35
  dimension "d180" = 142.24
  dimension "d181" = 142.24
  dimension "d182" = 142.24
  dimension "d183" = 6.35
  dimension "d184" = 58.42
  dimension "d185" = 6.35
  dimension "d186" = 58.42
  constraints: 48 end point, 12 parallel, 6 horizontal, 6 perpendicular, 3 point on line
  measures "d178" distance of L2.end L1.end
  measures "d179" distance of L1.end L0.end
  measures "d180" distance of L6.end L7.end
  measures "d181" distance of L12.end L11.end
  measures "d182" distance of L15.end L16.end
  measures "d183" distance of L14.end L15.end
  measures "d184" distance of L21.end L20.end
  measures "d185" distance of L20.end L19.end
  measures "d186" distance of L25.end L26.end
extrude "Extrusion22" add sketch "Sketch25" along normal blind 6.35
sketch "Sketch26" plane through (82.55, 0, -730.25) normal (0, 0, 1) x (1, 0, 0)
  line L0 (0, 0) -> (142.24, 0)
  line L1 (142.24, 0) -> (142.24, 6.35)
  line L2 (142.24, 6.35) -> (0, 6.35)
  line L3 (0, 6.35) -> (0, 0)
  line L4 (431.8, 0) -> (289.56, 0)
  line L5 (289.56, 0) -> (289.56, 6.35)
  line L6 (289.56, 6.35) -> (431.8, 6.35)
  line L7 (431.8, 6.35) -> (431.8, 0)
  line L8 (438.15, 0) -> (580.39, 0)
  line L9 (580.39, 0) -> (580.39, 6.35)
  line L10 (580.39, 6.35) -> (438.15, 6.35)
  line L11 (438.15, 6.35) -> (438.15, 0)
  line L12 (-6.35, 0) -> (1060.45, 0) projected
  line L13 (870.3653, 0) -> (728.1253, 0)
  line L14 (728.1253, 0) -> (728.1253, 6.35)
  line L15 (728.1253, 6.35) -> (870.3653, 6.35)
  line L16 (870.3653, 6.35) -> (870.3653, 0)
  line L17 (876.3, 0) -> (1054.1, 0) projected
  line L18 (876.3, 0) -> (934.72, 0)
  line L19 (934.72, 0) -> (934.72, 6.35)
  line L20 (934.72, 6.35) -> (876.3, 6.35)
  line L21 (876.3, 6.35) -> (876.3, 0)
  line L22 (1054.1, 0) -> (995.68, 0)
  line L23 (995.68, 0) -> (995.68, 6.35)
  line L24 (995.68, 6.35) -> (1054.1, 6.35)
  line L25 (1054.1, 6.35) -> (1054.1, 0)
  point P0 (-82.55, 0)
  point P1 (728.1253, 0)
  point P2 (934.72, 0)
  point P3 (995.68, 0)
  dimension "d189" = 142.24
  dimension "d190" = 6.35
  dimension "d191" = 142.24
  dimension "d192" = 6.35
  dimension "d193" = 142.24
  dimension "d194" = 142.24
  dimension "d195" = 6.35
  dimension "d196" = 58.42
  dimension "d197" = 58.42
  constraints: 48 end point, 12 parallel, 6 horizontal, 6 perpendicular, 2 point on line, 2 other
  measures "d189" distance of L2.end L1.end
  measures "d190" distance of L1.end L0.end
  measures "d191" distance of L5.end L6.end
  measures "d192" distance of L4.end L5.end
  measures "d193" distance of L10.end L9.end
  measures "d194" distance of L14.end L15.end
  measures "d195" distance of the line from the sketch origin of L15
  measures "d196" distance of L20.end L19.end
  measures "d197" distance of L23.end L24.end
extrude "Extrusion23" add sketch "Sketch26" along normal blind 6.35
body "Solid1"
